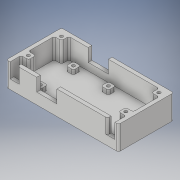
# Autodesk Inventor part: Link Adapter
Saved by Autodesk Inventor 2017 (Build 210142000, 142)
## iProperties
Created: 2020-09-04
Part Number: Link Adapter
Material: Generic
Document SubType Name: Modeling
Designer: Collin
Density: 1 g/cm^3
Appearance: Default
Author: Collin
## iProperties of the stored document Link Adapter_3DPrint.ipt
Created: 2022-10-02
Part Number: Link Adapter_3DPrint
Material: Generic
Document SubType Name: Modeling
Designer: Collin
Density: 1 g/cm^3
Appearance: Default
Author: Collin
Autodesk Inventor part; units mm, degrees
ref_plane "YZ Plane" through (0, 0, 0) normal (1, 0, 0) x (0, 1, 0)
ref_plane "XZ Plane" through (0, 0, 0) normal (0, 1, 0) x (-1, 0, 0)
ref_plane "XY Plane" through (0, 0, 0) normal (0, 0, 1) x (1, 0, 0)
sketch "Sketch1" plane through (0, 0, 0) normal (0, 1, 0) x (-1, 0, 0)
  line L0 (0, 0) -> (61, 0)
  line L1 (61, 0) -> (61, -30)
  line L2 (61, -30) -> (0, -30)
  line L3 (0, -30) -> (0, 0)
  dimension "d0" = 30
  dimension "d1" = 61
  constraints: 8 end point, 2 parallel, 1 horizontal, 1 perpendicular
  measures "d0" distance of L0.end L1.end
  measures "d1" distance of L1.end L2.end
extrude "Extrusion1" add sketch "Sketch1" along normal blind 13
sketch "Sketch4" plane through (0, 13, 0) normal (0, 1, 0) x (1, 0, 0)
  line L0 (-2, 2) -> (-59, 2)
  line L1 (-59, 2) -> (-59, 28)
  line L2 (-59, 28) -> (-2, 28)
  line L3 (-2, 28) -> (-2, 2)
  line L4 (-61, 0) -> (-61, 30) projected
  line L5 (0, 0) -> (-61, 0) projected
  line L6 (0, 30) -> (-61, 30) projected
  line L7 (0, 0) -> (0, 30) projected
  line L8 (-55, 24) -> (-59, 24)
  line L9 (-59, 24) -> (-59, 28)
  line L10 (-59, 28) -> (-55, 28)
  line L11 (-55, 28) -> (-55, 24)
  line L12 (-2, 28) -> (-6, 28)
  line L13 (-6, 28) -> (-6, 24)
  line L14 (-6, 24) -> (-2, 24)
  line L15 (-2, 24) -> (-2, 28)
  line L16 (-59, 6) -> (-55, 6)
  line L17 (-55, 6) -> (-55, 10)
  line L18 (-55, 10) -> (-59, 10)
  line L19 (-59, 10) -> (-59, 6)
  line L20 (-2, 6) -> (-6, 6)
  line L21 (-6, 6) -> (-6, 10)
  line L22 (-6, 10) -> (-2, 10)
  line L23 (-2, 10) -> (-2, 6)
  dimension "d18" = 2
  dimension "d19" = 2
  dimension "d20" = 2
  dimension "d21" = 2
  dimension "d26" = 4
  dimension "d27" = 4
  dimension "d30" = 4
  dimension "d31" = 4
  dimension "d53" = 4
  dimension "d54" = 4
  dimension "d57" = 0
  dimension "d61" = 6
  dimension "d139" = 4
  dimension "d140" = 4
  dimension "d141" = 0
  dimension "d142" = 6
  constraints: 40 end point, 10 parallel, 5 horizontal, 5 perpendicular
  measures "d18" distance between parallel lines of L4 L1
  measures "d19" distance between parallel lines of L5 L0
  measures "d20" distance between parallel lines of L6 L2
  measures "d21" distance between parallel lines of L7 L3
  measures "d26" distance of L8.start L8.end
  measures "d27" distance of L10.end L8.start
  measures "d30" distance of L12.end L13.end
  measures "d31" distance of L13.end L14.end
  measures "d53" distance of L17.end L18.end
  measures "d54" distance of L16.end L17.end
  measures "d57" distance between parallel lines of L1 L19
  measures "d61" distance between parallel lines of L5 L16
  measures "d139" distance of L20.end L21.end
  measures "d140" distance of L21.end L22.end
  measures "d141" distance between parallel lines of L23 L3
  measures "d142" distance between parallel lines of L5 L20
extrude "Extrusion3" cut sketch "Sketch4" against normal blind 11 contours L0 L1 L16 L17 L18 L8 L11 L2 L13 L14 L3 L22 L21 L20
sketch "Sketch5" plane through (-61, 0, 0) normal (0, 0, 1) x (1, 0, 0)
  line L0 (16.5, 13) -> (27.5, 13)
  line L1 (27.5, 13) -> (27.5, 6)
  line L2 (27.5, 6) -> (16.5, 6)
  line L3 (16.5, 6) -> (16.5, 13)
  line L4 (61, 0) -> (61, 13) projected
  line L5 (59, 13) -> (2, 13) projected
  line L6 (0, 0) -> (0, 13) projected
  point P0 (55, 13)
  point P1 (6, 13)
  dimension "d38" = 11
  dimension "d39" = 7
  dimension "d41" = 0
  dimension "d48" = 16.5
  constraints: 8 end point, 2 parallel, 1 horizontal, 1 perpendicular
  measures "d38" distance of L0.start L0.end
  measures "d39" distance of L0.end L1.end
  measures "d41" distance between parallel lines of L5 L0
  measures "d48" distance between parallel lines of L3 L6
extrude "Extrusion6" cut sketch "Sketch5" against normal through all
sketch "Sketch6" plane through (-61, 0, 0) normal (0, 0, 1) x (1, 0, 0)
  line L0 (55, 5) -> (59, 5)
  line L1 (59, 5) -> (59, 13)
  line L2 (59, 13) -> (55, 13)
  line L3 (55, 13) -> (55, 5)
  line L4 (61, 0) -> (61, 13) projected
  line L5 (27.5, 13) -> (61, 13) projected
  line L6 (61, 0) -> (0, 0) projected
  line L7 (2, 5) -> (6, 5)
  line L8 (6, 5) -> (6, 13)
  line L9 (6, 13) -> (2, 13)
  line L10 (2, 13) -> (2, 5)
  line L11 (0, 13) -> (16.5, 13) projected
  line L12 (0, 0) -> (0, 13) projected
  dimension "d45" = 6
  dimension "d47" = 0
  dimension "d50" = 4
  dimension "d63" = 5
  dimension "d64" = 0
  dimension "d65" = 4
  dimension "d66" = 5
  dimension "d67" = 6
  constraints: 16 end point, 4 parallel, 2 horizontal, 2 perpendicular
  measures "d45" distance between parallel lines of L4 L3
  measures "d47" distance between parallel lines of L5 L2
  measures "d50" distance of L0.start L0.end
  measures "d63" distance between parallel lines of L6 L0
  measures "d64" distance between parallel lines of L11 L9
  measures "d65" distance between parallel lines of L10 L8
  measures "d66" distance between parallel lines of L6 L7
  measures "d67" distance between parallel lines of L12 L8
extrude "Extrusion7" cut sketch "Sketch6" against normal blind 2
sketch "Sketch9" plane through (0, 2, 0) normal (0, 1, 0) x (1, 0, 0)
  line L0 (-55, 2) -> (-55, 0) projected
  line L1 (-55, 0) -> (-44.5, 0) projected
  line L2 (-44.5, 0) -> (-44.5, 2) projected
  line L3 (-44.5, 2) -> (-55, 2) projected
  line L4 (-6, 0) -> (-6, 2) projected
  line L5 (-6, 2) -> (-33.5, 2) projected
  line L6 (-33.5, 2) -> (-33.5, 0) projected
  line L7 (-33.5, 0) -> (-6, 0) projected
  line L8 (-44.5, 2) -> (-55, 2) projected
  line L9 (-50.5, 4) -> (-46.5, 4)
  line L10 (-46.5, 4) -> (-46.5, 8)
  line L11 (-46.5, 8) -> (-50.5, 8)
  line L12 (-50.5, 8) -> (-50.5, 4)
  line L13 (-46.5, 22) -> (-46.5, 26)
  line L14 (-46.5, 26) -> (-50.5, 26)
  line L15 (-50.5, 26) -> (-50.5, 22)
  line L16 (-50.5, 22) -> (-46.5, 22)
  line L17 (-27.5, 4) -> (-27.5, 8)
  line L18 (-27.5, 8) -> (-31.5, 8)
  line L19 (-31.5, 8) -> (-31.5, 4)
  line L20 (-31.5, 4) -> (-27.5, 4)
  line L21 (-27.5, 22) -> (-27.5, 26)
  line L22 (-27.5, 26) -> (-31.5, 26)
  line L23 (-31.5, 26) -> (-31.5, 22)
  line L24 (-31.5, 22) -> (-27.5, 22)
  line L25 (-55, 28) -> (-6, 28) projected
  line L26 (-44.5, 30) -> (-61, 30) projected
  dimension "d202" = 4
  dimension "d203" = 4
  dimension "d204" = 2
  dimension "d205" = 2
  dimension "d208" = 18
  dimension "d211" = 19
  dimension "d231" = 2
  dimension "d232" = 30
  dimension "d233" = 2
  constraints: 32 end point, 2 collinear, 2 horizontal, 2 parallel, 1 perpendicular, 1 vertical, 22 other
  measures "d202" distance of L10.end L11.end
  measures "d203" distance of L11.end L9.start
  measures "d204" distance between parallel lines of L2 L10
  measures "d205" distance between parallel lines of L3 L9
  measures "d208" distance of L9.end L13.start
  measures "d211" distance of L9.end L17.start
  measures "d231" distance between parallel lines of L25 L14
  measures "d232" distance between parallel lines of L26 L1
  measures "d233" distance between parallel lines of L6 L19
extrude "Extrusion8" add sketch "Sketch9" along normal blind 2.4 contours L12 L11 L10 L9 | L16 L15 L14 L13 | L20 L19 L18 L17 | L24 L23 L22 L21
chamfer "Chamfer2" distance 1 angle 45 2 edges at (-55, 9, 0) (-6, 9, 0)
fillet "Fillet1" radius 1 34 edges at (-61, 6.5, 0) (0, 6.5, 0) (0, 6.5, -30) (-61, 6.5, -30) (-55, 7.5, -24) (-59, 7.5, -24) (-55, 7.5, -28) (-59, 7.5, -6) (-55, 7.5, -6) (-55, 7.5, -10) (-59, 7.5, -10) (-2, 7.5, -6) (-6, 7.5, -6) (-6, 7.5, -10) (-2, 7.5, -10) (-6, 7.5, -24) (-2, 7.5, -24) (-6, 7.5, -28) (-31.5, 3.2, -22) (-27.5, 3.2, -22) (-46.5, 3.2, -22) (-50.5, 3.2, -22) (-46.5, 3.2, -8) (-50.5, 3.2, -8) (-31.5, 3.2, -8) (-27.5, 3.2, -8) (-46.5, 3.2, -4) (-50.5, 3.2, -4) (-31.5, 3.2, -4) (-27.5, 3.2, -4) (-50.5, 3.2, -26) (-46.5, 3.2, -26) (-31.5, 3.2, -26) (-27.5, 3.2, -26)
sketch "Sketch7" plane through (0, 13, 0) normal (0, 1, 0) x (1, 0, 0)
  circle A0 centre (-57, 26) radius 0.75
  circle A1 centre (-4, 26) radius 0.75
  circle A2 centre (-57, 8) radius 0.75
  line L0 (-55, 24) -> (-55, 28) projected
  line L1 (-59, 24) -> (-55, 24) projected
  line L2 (-6, 24) -> (-2, 24) projected
  line L3 (-6, 28) -> (-6, 24) projected
  line L4 (-55, 6) -> (-55, 10) projected
  line L5 (-59, 6) -> (-55, 6) projected
  circle A3 centre (-4, 8) radius 0.75
  line L6 (-6, 10) -> (-6, 6) projected
  line L7 (-6, 6) -> (-2, 6) projected
  point P0 (0, 0)
  dimension "d68" = 1.5
  dimension "d70" = 1.5
  dimension "d71" = 1.5
  dimension "d72" = 2
  dimension "d73" = 2
  dimension "d74" = 2
  dimension "d75" = 2
  dimension "d78" = 2
  dimension "d79" = 2
  dimension "d143" = 1.5
  dimension "d145" = 2
  dimension "d146" = 2
  constraints: 4 centre point
  measures "d68" diameter of A2
  measures "d70" diameter of A1
  measures "d71" diameter of A0
  measures "d72" distance from line of L0 A0.centre
  measures "d73" distance from line of L1 A0.centre
  measures "d74" distance from line of L2 A1.centre
  measures "d75" distance from line of L3 A1.centre
  measures "d78" distance from line of L4 A2.centre
  measures "d79" distance from line of L5 A2.centre
  measures "d143" diameter of A3
  measures "d145" distance from line of A3.centre L6
  measures "d146" distance from line of L7 A3.centre
hole "Hole1" at (-57, 13, -26) at (-4, 13, -26) at (-57, 13, -8) at (-4, 13, -8) direction (0, -1, 0) diameter 1.7 depth 10
sketch "Sketch14" plane through (0, 4.4, 0) normal (0, 1, 0) x (1, 0, 0)
  line L0 (-50.5, 7) -> (-50.5, 5) projected
  line L1 (-47.5, 8) -> (-49.5, 8) projected
  point P0 (0, 0)
  point P1 (-48.5, 6)
  point P2 (-49, 3)
  point P3 (-48.5, 24)
  point P4 (-29.5, 6)
  point P5 (-29.5, 24)
  point P6 (-49, 4)
  dimension "d214" = 2
  dimension "d215" = 2
  dimension "d218" = 18
  dimension "d221" = 19
  constraints: 1 horizontal, 1 vertical alignment, 3 other
  measures "d215" distance from line of L1 point (-48.5, 6)
  measures "d218" distance of point (-48.5, 6) point (-48.5, 24)
  measures "d221" distance of point (-48.5, 6) point (-29.5, 6)
hole "Hole4" at (-48.5, 4.4, -6) at (-48.5, 4.4, -24) at (-29.5, 4.4, -6) at (-29.5, 4.4, -24) direction (0, -1, 0) diameter 1.7 depth 2 tip angle 118
body "Solid1"
